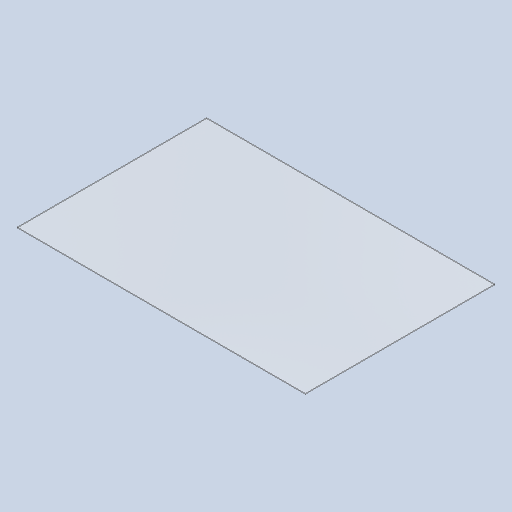
# Autodesk Inventor part: Base
Saved by Autodesk Inventor 2025.1 (Build 291241000, 241)
## iProperties
Created: 2024-09-06
Part Number: Base
Material: Acrylic
Document SubType Name: Modeling
Designer: joser
Density: 1.188 g/cm^3
Appearance: Transparent - Clear
Author: joser
Autodesk Inventor part; units mm, degrees
ref_plane "YZ Plane" through (0, 0, 0) normal (1, 0, 0) x (0, 1, 0)
ref_plane "XZ Plane" through (0, 0, 0) normal (0, 1, 0) x (-1, 0, 0)
ref_plane "XY Plane" through (0, 0, 0) normal (0, 0, 1) x (1, 0, 0)
sketch "Sketch1" plane through (0, 0, 0) normal (0, 1, 0) x (-1, 0, 0)
  line L0 (-584, 384) -> (584, 384)
  line L1 (584, 384) -> (584, -384)
  line L2 (584, -384) -> (-584, -384)
  line L3 (-584, -384) -> (-584, 384)
  line L4 (-584, 384) -> (584, -384) construction
  line L5 (584, 384) -> (-584, -384) construction
  point P0 (0, 0)
  dimension "d0" = 1168
  dimension "d1" = 768
  constraints: 12 end point, 2 midpoint, 2 parallel, 1 horizontal, 1 perpendicular
  measures "d0" distance of L1.end L2.end
  measures "d1" distance of L0.end L1.end
extrude "Extrusion1" add sketch "Sketch1" along normal mid plane 3
body "Solid1"
